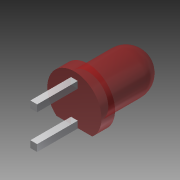
# Autodesk Inventor part: LED3mm
Saved by Autodesk Inventor 2014 SP1 (Build 180222100, 222)
## iProperties
Created: 2016-03-19
Part Number: LED3mm
Material: Generic
Document SubType Name: Modeling
Designer: Tyler
Density: 1 g/cm^3
Appearance: Dark Red
Author: Tyler
Autodesk Inventor part; units mm, degrees
ref_plane "YZ Plane" through (0, 0, 0) normal (1, 0, 0) x (0, 1, 0)
ref_plane "XZ Plane" through (0, 0, 0) normal (0, 1, 0) x (-1, 0, 0)
ref_plane "XY Plane" through (0, 0, 0) normal (0, 0, 1) x (1, 0, 0)
sketch "Sketch1" plane through (0, 0, 0) normal (0, 0, 1) x (1, 0, 0)
  arc A0 (1.5, 3.8) -> (0, 5.3) centre (0, 3.8) ccw
  line L0 (1.5, 3.8) -> (1.5, 1)
  line L1 (1.5, 1) -> (2, 1)
  line L2 (2, 1) -> (2, 0)
  line L3 (2, 0) -> (0, 0)
  line L4 (0, 0) -> (0, 5.3)
  point P0 (0, 0)
  dimension "d0" = 3
  dimension "d1" = 2
  dimension "d2" = 1
  dimension "d3" = 5.3
  dimension "d4" = 0
  dimension "d5" = 0
  dimension "d6" = 0
  constraints: 10 end point, 3 parallel, 2 point on circle, 1 centre point, 1 perpendicular, 1 tangent, 1 vertical
  measures "d0" diameter of A0
  measures "d1" distance between parallel lines of L4 L2
  measures "d2" distance of L1.end L2.end
  measures "d3" distance from line of L4.end L3
  measures "d4" distance from line of point (0, 0) L3
  measures "d5" distance from line of point (0, 0) L4
  measures "d6" distance from line of L4 A0.centre
revolve "Revolution1" add sketch "Sketch1" angle 360 about axis through (0, 0, 0) along (0, 1, 0)
sketch "Sketch2" plane through (0, 0, 0) normal (0, 1, 0) x (-1, 0, 0)
  line L0 (-2.5, -4.5) -> (2.5, -4.5)
  line L1 (2.5, -4.5) -> (2.5, -1.5)
  line L2 (2.5, -1.5) -> (-2.5, -1.5)
  line L3 (-2.5, -1.5) -> (-2.5, -4.5)
  line L4 (-2.5, -4.5) -> (2.5, -1.5) construction
  line L5 (2.5, -4.5) -> (-2.5, -1.5) construction
  point P0 (0, 0)
  point P1 (0, -3)
  dimension "d8" = 1.5
  dimension "d9" = 5
  dimension "d10" = 3
  dimension "d12" = 2.5
  constraints: 12 end point, 2 midpoint, 2 parallel, 1 horizontal, 1 perpendicular
  measures "d8" distance from line of L2 point (0, 0)
  measures "d9" distance of L1.end L2.end
  measures "d10" distance of L2.end L0.start
  measures "d12" distance from line of point (0, 0) L1
extrude "Extrusion1" cut sketch "Sketch2" along normal blind 10
sketch "Sketch3" plane through (0, 0, 0) normal (0, -1, 0) x (1, 0, 0)
  arc A0 (1.3229, -1.5) -> (-1.3229, -1.5) centre (0, 0) ccw projected
  line L0 (-0.25, -1.52) -> (0.25, -1.52)
  line L1 (0.25, -1.52) -> (0.25, -1.02)
  line L2 (0.25, -1.02) -> (-0.25, -1.02)
  line L3 (-0.25, -1.02) -> (-0.25, -1.52)
  line L4 (-0.25, -1.52) -> (0.25, -1.02) construction
  line L5 (0.25, -1.52) -> (-0.25, -1.02) construction
  line L6 (-0.25, 1.02) -> (0.25, 1.02)
  line L7 (0.25, 1.02) -> (0.25, 1.52)
  line L8 (0.25, 1.52) -> (-0.25, 1.52)
  line L9 (-0.25, 1.52) -> (-0.25, 1.02)
  line L10 (-0.25, 1.02) -> (0.25, 1.52) construction
  line L11 (0.25, 1.02) -> (-0.25, 1.52) construction
  point P0 (0, -1.27)
  point P1 (0, 1.27)
  dimension "d15" = 0.5
  dimension "d16" = 0.5
  dimension "d17" = 0.5
  dimension "d18" = 0.5
  dimension "d19" = 2.54
  dimension "d20" = 1.27
  constraints: 24 end point, 4 midpoint, 4 parallel, 2 horizontal, 2 perpendicular
  measures "d15" distance of L2.end L1.end
  measures "d16" distance of L1.end L0.end
  measures "d17" distance of L8.end L7.end
  measures "d18" distance of L7.end L6.end
  measures "d19" distance of point (0, -1.27) point (0, 1.27)
  measures "d20" distance of A0.centre point (0, 1.27)
extrude "Extrusion2" add sketch "Sketch3" along normal blind 3
equation "\"d12\" = 0.5 * d9"
equation "\"d20\" = 0.5 * d19"
body "Solid1"
